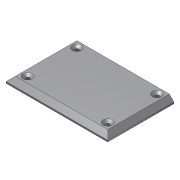
# Autodesk Inventor part: Tampa - Chip kick
Saved by Autodesk Inventor 2011 (Build 150239000, 239)
## iProperties
Created: 2011-04-10
Part Number: Tampa - Chip kick
Document SubType Name: Modeling
Designer: Milton
Density: 1 g/cm^3
Author: Milton
Autodesk Inventor part; units mm, degrees
ref_plane "YZ Plane" through (0, 0, 0) normal (1, 0, 0) x (0, 1, 0)
ref_plane "XZ Plane" through (0, 0, 0) normal (0, 1, 0) x (-1, 0, 0)
ref_plane "XY Plane" through (0, 0, 0) normal (0, 0, 1) x (1, 0, 0)
sketch "Sketch1" plane through (0, 0, 0) normal (0, 0, 1) x (1, 0, 0)
  circle A0 centre (69.1044, 19.9218) radius 3 projected
  circle A1 centre (69.1044, -7.6264) radius 3 projected
  circle A2 centre (47.2099, -41.3409) radius 3 projected
  circle A3 centre (-47.265, -41.3409) radius 3 projected
  circle A4 centre (-69.1594, -7.6264) radius 3 projected
  circle A5 centre (-69.1594, 19.9218) radius 3 projected
  circle A6 centre (47.2099, 53.6364) radius 3 projected
  circle A7 centre (-47.265, 53.6364) radius 3 projected
  line L0 (78.9735, 4.1477) -> (78.9735, 8.1477) projected
  line L1 (78.9735, 8.1477) -> (82.9735, 8.1477) projected
  line L2 (82.9735, 8.1477) -> (82.9735, 4.1477) projected
  line L3 (82.9735, 4.1477) -> (78.9735, 4.1477) projected
  line L4 (-83.0286, 4.1477) -> (-83.0286, 8.1477) projected
  line L5 (-83.0286, 8.1477) -> (-79.0286, 8.1477) projected
  line L6 (-79.0286, 8.1477) -> (-79.0286, 4.1477) projected
  line L7 (-79.0286, 4.1477) -> (-83.0286, 4.1477) projected
  line L8 (70.8258, 23.6974) -> (40.6226, 70.2061) projected
  line L9 (40.6226, 70.2061) -> (26.9729, 70.2061) projected
  line L10 (26.9729, 70.2061) -> (26.9729, 30.2061) projected
  line L11 (26.9729, 30.2061) -> (22.9729, 30.2061) projected
  line L12 (22.9729, 30.2061) -> (22.9729, -12.7939) projected
  line L13 (22.9729, -12.7939) -> (-23.0279, -12.7939) projected
  line L14 (-23.0279, -12.7939) -> (-23.0279, 30.2061) projected
  line L15 (-23.0279, 30.2061) -> (-27.0279, 30.2061) projected
  line L16 (-27.0279, 30.2061) -> (-27.0279, 70.2061) projected
  line L17 (-27.0279, 70.2061) -> (-40.6777, 70.2061) projected
  line L18 (-40.6777, 70.2061) -> (-70.8809, 23.6974) projected
  arc A8 (-73.3969, 22.3313) -> (-70.8809, 23.6974) centre (-73.3969, 25.3313) ccw projected
  line L19 (-73.3969, 22.3313) -> (-82.8214, 22.3313) projected
  arc A9 (-82.8214, 22.3313) -> (-84.7927, 20.669) centre (-82.8214, 20.3313) ccw projected
  arc A10 (-84.7927, 20.669) -> (-84.7927, -8.3735) centre (-0.0275, 6.1477) ccw projected
  arc A11 (-84.7927, -8.3735) -> (-82.8214, -10.0358) centre (-82.8214, -8.0358) ccw projected
  line L20 (-82.8214, -10.0358) -> (-73.3969, -10.0358) projected
  arc A12 (-70.8809, -11.4019) -> (-73.3969, -10.0358) centre (-73.3969, -13.0358) ccw projected
  line L21 (-70.8809, -11.4019) -> (-44.8786, -51.4419) projected
  arc A13 (-44.6539, -54.2961) -> (-44.8786, -51.4419) centre (-47.3946, -53.0758) ccw projected
  line L22 (-44.6539, -54.2961) -> (-48.4872, -62.9058) projected
  arc A14 (-48.4872, -62.9058) -> (-47.7705, -65.3828) centre (-46.6602, -63.7193) ccw projected
  arc A15 (-47.7705, -65.3828) -> (47.7154, -65.3828) centre (-0.0275, 6.1477) ccw projected
  arc A16 (47.7154, -65.3828) -> (48.4322, -62.9058) centre (46.6051, -63.7193) ccw projected
  line L23 (48.4322, -62.9058) -> (44.5989, -54.2961) projected
  arc A17 (44.8235, -51.4419) -> (44.5989, -54.2961) centre (47.3395, -53.0758) ccw projected
  line L24 (44.8235, -51.4419) -> (71.7129, -10.0358) projected
  line L25 (71.7129, -10.0358) -> (82.7663, -10.0358) projected
  arc A18 (82.7663, -10.0358) -> (84.7376, -8.3735) centre (82.7663, -8.0358) ccw projected
  arc A19 (84.7376, -8.3735) -> (84.7376, 20.669) centre (-0.0275, 6.1477) ccw projected
  arc A20 (84.7376, 20.669) -> (82.7663, 22.3313) centre (82.7663, 20.3313) ccw projected
  line L26 (82.7663, 22.3313) -> (73.3418, 22.3313) projected
  arc A21 (70.8258, 23.6974) -> (73.3418, 22.3313) centre (73.3418, 25.3313) ccw projected
  line L27 (32.9729, 30.2061) -> (-33.0279, 30.2061)
  line L28 (-33.0279, 30.2061) -> (-33.0279, -12.7939)
  line L29 (-33.0279, -12.7939) -> (32.9729, -12.7939)
  line L30 (32.9729, -12.7939) -> (32.9729, 30.2061)
  point P0 (0, 0)
  dimension "d0" = 10
  dimension "d1" = 10
  constraints: 8 end point, 3 parallel, 1 perpendicular
  measures "d0" distance between parallel lines of L12 L30
  measures "d1" distance between parallel lines of L28 L14
extrude "Extrusion1" add sketch "Sketch1" along normal blind 4 contours L27 L30 L29 L12 L11 | L12 L13 L14 L27 | L14 L29 L28 L27 L15
chamfer "Chamfer1" distance 3 angle 45 3 edges at (32.9729, 8.7061, 4) (-33.0279, 8.7061, 4) (-0.0275, -12.7939, 4)
sketch "Sketch2" plane through (0, 0, 4) normal (0, 0, 1) x (1, 0, 0)
  line L0 (-30.0279, -9.7939) -> (-30.0279, 30.2061) projected
  line L1 (29.9729, -9.7939) -> (-30.0279, -9.7939) projected
  line L2 (29.9729, 30.2061) -> (29.9729, -9.7939) projected
  line L3 (-30.0279, 30.2061) -> (29.9729, 30.2061) projected
  circle A0 centre (-26.0279, 26.2061) radius 1.5
  circle A1 centre (25.9729, 26.2061) radius 1.5
  circle A2 centre (-26.0279, -5.7939) radius 1.5
  circle A3 centre (25.9729, -5.7939) radius 1.5
  point P0 (0, 0)
  dimension "d7" = 3
  dimension "d8" = 3
  dimension "d9" = 3
  dimension "d10" = 3
  dimension "d11" = 4
  dimension "d12" = 4
  dimension "d13" = 4
  dimension "d14" = 4
  dimension "d15" = 4
  dimension "d16" = 4
  dimension "d17" = 4
  dimension "d18" = 4
  constraints: 4 centre point
  measures "d7" diameter of A0
  measures "d8" diameter of A1
  measures "d9" diameter of A2
  measures "d10" diameter of A3
  measures "d11" distance from line of L0 A0.centre
  measures "d12" distance from line of L3 A0.centre
  measures "d13" distance from line of L3 A1.centre
  measures "d14" distance from line of L2 A1.centre
  measures "d15" distance from line of L0 A2.centre
  measures "d16" distance from line of L1 A2.centre
  measures "d17" distance from line of L2 A3.centre
  measures "d18" distance from line of L1 A3.centre
hole "Hole1" at (25.9729, 26.2061, 4) at (25.9729, -5.7939, 4) at (-26.0279, 26.2061, 4) at (-26.0279, -5.7939, 4) direction (0, 0, -1) diameter 3 depth 8 tip angle 118 countersink diameter 6 countersink angle 90
body "Solid1"
